Autodesk Inventor part; units mm, degrees
(part 11 of 16)
  spline S66 degree 3 poles (-38.2269, 71.8487) (-38.3811, 71.843) (-38.5356, 71.8444) (-38.6895, 71.8542) (-38.7353, 71.8572) (-38.781, 71.8608) (-38.8267, 71.8653) (-38.8695, 71.8695) (-38.9124, 71.8744) (-38.9551, 71.88) (-38.995, 71.8853) (-39.0349, 71.8912) (-39.0747, 71.8978) (-39.1117, 71.9039) (-39.1486, 71.9107) (-39.1854, 71.9181) (-39.2195, 71.9249) (-39.2534, 71.9323) (-39.2872, 71.9403) (-39.3183, 71.9476) (-39.3493, 71.9555) (-39.3802, 71.9639) (-39.4084, 71.9715) (-39.4364, 71.9796) (-39.4643, 71.9882) (-39.4895, 71.996) (-39.5146, 72.0042) (-39.5396, 72.0128) (-39.562, 72.0205) (-39.5843, 72.0284) (-39.6062, 72.0371) (-39.6255, 72.0447) (-39.6445, 72.0529) (-39.6642, 72.0604) (-39.7009, 72.0743) (-39.7403, 72.0857) (-39.7695, 72.1099) (-39.7917, 72.1282) (-39.8081, 72.1539) (-39.8266, 72.177) (-39.8422, 72.1963) (-39.8592, 72.2138) (-39.8762, 72.2316) (-39.8928, 72.2488) (-39.9093, 72.2662) (-39.9262, 72.2833) (-39.9426, 72.2999) (-39.9594, 72.3162) (-39.9764, 72.3322) (-39.9929, 72.3478) (-40.0097, 72.3632) (-40.0267, 72.3783) (-40.0434, 72.393) (-40.0602, 72.4074) (-40.0773, 72.4215) (-40.094, 72.4353) (-40.1109, 72.4488) (-40.128, 72.462) (-40.1447, 72.4749) (-40.1617, 72.4875) (-40.1789, 72.4998) (-40.1956, 72.5117) (-40.2126, 72.5234) (-40.2298, 72.5347) (-40.2466, 72.5458) (-40.2636, 72.5566) (-40.2809, 72.567) (-40.2977, 72.5772) (-40.3148, 72.587) (-40.3321, 72.5965) (-40.349, 72.6058) (-40.3661, 72.6147) (-40.3835, 72.6232) (-40.4005, 72.6316) (-40.4177, 72.6396) (-40.4351, 72.6472) (-40.4522, 72.6547) (-40.4695, 72.6617) (-40.487, 72.6683) (-40.5042, 72.6749) (-40.5217, 72.681) (-40.5393, 72.6866) (-40.5567, 72.6922) (-40.5743, 72.6973) (-40.5921, 72.7019) (-40.6097, 72.7064) (-40.6276, 72.7105) (-40.6455, 72.714) (-40.6635, 72.7175) (-40.6815, 72.7204) (-40.6997, 72.7228) (-40.718, 72.7251) (-40.7364, 72.7268) (-40.7548, 72.7279) (-40.7735, 72.7289) (-40.7923, 72.7293) (-40.811, 72.7289) (-40.8301, 72.7285) (-40.8492, 72.7273) (-40.8682, 72.7254) (-40.8877, 72.7233) (-40.9072, 72.7204) (-40.9265, 72.7166) (-40.9463, 72.7127) (-40.966, 72.7078) (-40.9854, 72.702) (-41.0054, 72.6959) (-41.0252, 72.6888) (-41.0445, 72.6807) (-41.0644, 72.6722) (-41.0839, 72.6627) (-41.1028, 72.6521) (-41.1222, 72.6411) (-41.141, 72.629) (-41.159, 72.6157) (-41.1774, 72.6022) (-41.1949, 72.5874) (-41.2116, 72.5718) (-41.2234, 72.5607) (-41.2348, 72.5491) (-41.2461, 72.5373) (-41.3001, 72.481) (-41.3504, 72.4211) (-41.4042, 72.3646) (-41.458, 72.3081) (-41.5152, 72.2549) (-41.5689, 72.1981) (-41.58, 72.1863) (-41.591, 72.1744) (-41.6016, 72.162) (-41.6164, 72.1446) (-41.6302, 72.1263) (-41.6429, 72.1073) (-41.6552, 72.0887) (-41.6664, 72.0693) (-41.6764, 72.0494) (-41.686, 72.03) (-41.6946, 72.0101) (-41.702, 71.9897) (-41.7092, 71.97) (-41.7154, 71.95) (-41.7204, 71.9297) (-41.7253, 71.91) (-41.7292, 71.8901) (-41.7321, 71.8701) (-41.735, 71.8506) (-41.7369, 71.8311) (-41.738, 71.8115) (-41.739, 71.7924) (-41.7392, 71.7732) (-41.7387, 71.7541) (-41.7381, 71.7354) (-41.7368, 71.7167) (-41.7349, 71.6981) (-41.7329, 71.6797) (-41.7303, 71.6614) (-41.727, 71.6433) (-41.7238, 71.6253) (-41.72, 71.6073) (-41.7156, 71.5896) (-41.7112, 71.5718) (-41.7063, 71.5542) (-41.7008, 71.5368) (-41.6954, 71.5193) (-41.6894, 71.502) (-41.683, 71.4848) (-41.6765, 71.4675) (-41.6695, 71.4504) (-41.6621, 71.4335) (-41.6547, 71.4164) (-41.6468, 71.3994) (-41.6385, 71.3827) (-41.63, 71.3657) (-41.6212, 71.3489) (-41.612, 71.3324) (-41.6026, 71.3155) (-41.5928, 71.2988) (-41.5827, 71.2824) (-41.5724, 71.2656) (-41.5617, 71.249) (-41.5507, 71.2327) (-41.5395, 71.216) (-41.5279, 71.1995) (-41.516, 71.1833) (-41.5038, 71.1666) (-41.4913, 71.1503) (-41.4785, 71.1341) (-41.4654, 71.1176) (-41.452, 71.1013) (-41.4383, 71.0852) (-41.4243, 71.0687) (-41.41, 71.0525) (-41.3954, 71.0366) (-41.3804, 71.0202) (-41.3652, 71.0041) (-41.3497, 70.9882) (-41.3337, 70.9719) (-41.3176, 70.9559) (-41.3011, 70.9401) (-41.2843, 70.924) (-41.2672, 70.908) (-41.2498, 70.8924) (-41.232, 70.8764) (-41.2138, 70.8608) (-41.1957, 70.8451) (-41.1772, 70.829) (-41.1588, 70.8128) (-41.1387, 70.7983) (-41.1147, 70.7809) (-41.0883, 70.7658) (-41.0689, 70.7446) (-41.0433, 70.7165) (-41.03, 70.6778) (-41.0143, 70.6418) (-41.0058, 70.6225) (-40.9967, 70.6039) (-40.9881, 70.585) (-40.9783, 70.5636) (-40.9693, 70.5417) (-40.9606, 70.5197) (-40.9508, 70.4951) (-40.9413, 70.4705) (-40.9323, 70.4457) (-40.9223, 70.4183) (-40.9128, 70.3907) (-40.9038, 70.3629) (-40.8939, 70.3325) (-40.8845, 70.302) (-40.8756, 70.2713) (-40.866, 70.2379) (-40.8569, 70.2043) (-40.8484, 70.1706) (-40.8392, 70.1343) (-40.8306, 70.0977) (-40.8227, 70.061) (-40.8141, 70.0217) (-40.8062, 69.9821) (-40.799, 69.9425) (-40.7913, 69.9001) (-40.7843, 69.8576) (-40.778, 69.815) (-40.7712, 69.7696) (-40.7653, 69.7241) (-40.7601, 69.6785) (-40.7427, 69.5253) (-40.7337, 69.371) (-40.7317, 69.2168) knots 0 0 0 0 0.065113 0.065113 0.065113 0.084473 0.084473 0.084473 0.102659 0.102659 0.102659 0.119672 0.119672 0.119672 0.135512 0.135512 0.135512 0.150178 0.150178 0.150178 0.163672 0.163672 0.163672 0.175991 0.175991 0.175991 0.187138 0.187138 0.187138 0.197111 0.197111 0.197111 0.205911 0.205911 0.205911 0.222284 0.222284 0.222284 0.234681 0.234681 0.234681 0.24506 0.24506 0.24506 0.255176 0.255176 0.255176 0.265035 0.265035 0.265035 0.274643 0.274643 0.274643 0.284008 0.284008 0.284008 0.293139 0.293139 0.293139 0.302047 0.302047 0.302047 0.310743 0.310743 0.310743 0.319241 0.319241 0.319241 0.327556 0.327556 0.327556 0.335706 0.335706 0.335706 0.343713 0.343713 0.343713 0.351599 0.351599 0.351599 0.359392 0.359392 0.359392 0.367126 0.367126 0.367126 0.374835 0.374835 0.374835 0.382562 0.382562 0.382562 0.390352 0.390352 0.390352 0.398256 0.398256 0.398256 0.406325 0.406325 0.406325 0.41461 0.41461 0.41461 0.423156 0.423156 0.423156 0.431994 0.431994 0.431994 0.441132 0.441132 0.441132 0.450548 0.450548 0.450548 0.460189 0.460189 0.460189 0.467051 0.467051 0.467051 0.5 0.5 0.5 0.532949 0.532949 0.532949 0.539811 0.539811 0.539811 0.549452 0.549452 0.549452 0.558868 0.558868 0.558868 0.568006 0.568006 0.568006 0.576844 0.576844 0.576844 0.58539 0.58539 0.58539 0.593675 0.593675 0.593675 0.601744 0.601744 0.601744 0.609648 0.609648 0.609648 0.617438 0.617438 0.617438 0.625165 0.625165 0.625165 0.632874 0.632874 0.632874 0.640608 0.640608 0.640608 0.648401 0.648401 0.648401 0.656287 0.656287 0.656287 0.664294 0.664294 0.664294 0.672444 0.672444 0.672444 0.680759 0.680759 0.680759 0.689257 0.689257 0.689257 0.697953 0.697953 0.697953 0.706861 0.706861 0.706861 0.715992 0.715992 0.715992 0.725357 0.725357 0.725357 0.734965 0.734965 0.734965 0.744824 0.744824 0.744824 0.75494 0.75494 0.75494 0.765319 0.765319 0.765319 0.777716 0.777716 0.777716 0.794089 0.794089 0.794089 0.802889 0.802889 0.802889 0.812862 0.812862 0.812862 0.824009 0.824009 0.824009 0.836328 0.836328 0.836328 0.849822 0.849822 0.849822 0.864488 0.864488 0.864488 0.880328 0.880328 0.880328 0.897341 0.897341 0.897341 0.915527 0.915527 0.915527 0.934887 0.934887 0.934887 1 1 1 1
  arc A268 (-38.2269, 71.8487) -> (-37.7508, 72.7226) centre (-45.7832, 76.5321) ccw
  spline S67 degree 3 poles (-36.8976, 76.2543) (-37.0282, 76.1723) (-37.1627, 76.0963) (-37.3009, 76.0278) (-37.342, 76.0075) (-37.3835, 75.9878) (-37.4252, 75.9688) (-37.4645, 75.951) (-37.504, 75.9338) (-37.5438, 75.9173) (-37.581, 75.9019) (-37.6185, 75.8871) (-37.6563, 75.8729) (-37.6914, 75.8598) (-37.7267, 75.8471) (-37.7623, 75.8351) (-37.7952, 75.824) (-37.8283, 75.8135) (-37.8616, 75.8035) (-37.8922, 75.7943) (-37.923, 75.7856) (-37.9539, 75.7774) (-37.9821, 75.77) (-38.0104, 75.7629) (-38.0389, 75.7565) (-38.0646, 75.7506) (-38.0905, 75.7452) (-38.1164, 75.7401) (-38.1396, 75.7355) (-38.1629, 75.7312) (-38.1862, 75.7278) (-38.2068, 75.7248) (-38.2273, 75.7224) (-38.2481, 75.719) (-38.2869, 75.7127) (-38.3266, 75.7029) (-38.3641, 75.7092) (-38.3924, 75.714) (-38.4194, 75.728) (-38.4471, 75.7388) (-38.4702, 75.7477) (-38.4938, 75.7544) (-38.5173, 75.7612) (-38.5403, 75.7679) (-38.5633, 75.7747) (-38.5864, 75.781) (-38.609, 75.7872) (-38.6316, 75.7929) (-38.6543, 75.7983) (-38.6765, 75.8035) (-38.6987, 75.8085) (-38.721, 75.813) (-38.7428, 75.8174) (-38.7646, 75.8215) (-38.7864, 75.8252) (-38.8078, 75.8288) (-38.8292, 75.8321) (-38.8506, 75.8349) (-38.8715, 75.8377) (-38.8925, 75.8401) (-38.9135, 75.8422) (-38.934, 75.8442) (-38.9546, 75.8458) (-38.9751, 75.847) (-38.9952, 75.8482) (-39.0153, 75.849) (-39.0355, 75.8494) (-39.0552, 75.8498) (-39.0749, 75.8498) (-39.0946, 75.8493) (-39.1139, 75.8489) (-39.1332, 75.8481) (-39.1524, 75.8468) (-39.1714, 75.8455) (-39.1903, 75.8439) (-39.2091, 75.8417) (-39.2277, 75.8397) (-39.2462, 75.8371) (-39.2646, 75.8341) (-39.2828, 75.8311) (-39.301, 75.8277) (-39.319, 75.8238) (-39.3369, 75.8199) (-39.3547, 75.8155) (-39.3724, 75.8106) (-39.39, 75.8057) (-39.4075, 75.8003) (-39.4247, 75.7944) (-39.442, 75.7885) (-39.4592, 75.782) (-39.4761, 75.7749) (-39.4931, 75.7678) (-39.5099, 75.7601) (-39.5264, 75.7517) (-39.5431, 75.7433) (-39.5595, 75.7342) (-39.5755, 75.7246) (-39.5919, 75.7147) (-39.6078, 75.7041) (-39.6233, 75.6929) (-39.6392, 75.6813) (-39.6546, 75.6691) (-39.6694, 75.6562) (-39.6846, 75.6429) (-39.6992, 75.6288) (-39.7131, 75.614) (-39.7274, 75.5988) (-39.741, 75.5827) (-39.7536, 75.566) (-39.7667, 75.5488) (-39.7788, 75.5308) (-39.7898, 75.5121) (-39.8012, 75.4929) (-39.8114, 75.473) (-39.8203, 75.4526) (-39.8295, 75.4316) (-39.8373, 75.4101) (-39.8439, 75.3882) (-39.8486, 75.3726) (-39.8526, 75.3569) (-39.8565, 75.3411) (-39.8751, 75.2653) (-39.8888, 75.1883) (-39.9071, 75.1125) (-39.9254, 75.0366) (-39.9484, 74.9619) (-39.9665, 74.886) (-39.9702, 74.8702) (-39.9738, 74.8543) (-39.9767, 74.8383) (-39.9808, 74.8158) (-39.9837, 74.7931) (-39.9852, 74.7703) (-39.9865, 74.748) (-39.9865, 74.7257) (-39.9852, 74.7034) (-39.9839, 74.6818) (-39.9813, 74.6602) (-39.9776, 74.6389) (-39.974, 74.6182) (-39.9693, 74.5978) (-39.9635, 74.5777) (-39.9579, 74.5582) (-39.9513, 74.539) (-39.9438, 74.5202) (-39.9366, 74.502) (-39.9285, 74.4841) (-39.9196, 74.4665) (-39.9109, 74.4495) (-39.9016, 74.4328) (-39.8915, 74.4165) (-39.8817, 74.4006) (-39.8712, 74.385) (-39.8602, 74.3699) (-39.8493, 74.355) (-39.8379, 74.3405) (-39.826, 74.3264) (-39.8142, 74.3124) (-39.802, 74.2988) (-39.7893, 74.2856) (-39.7766, 74.2724) (-39.7635, 74.2596) (-39.7501, 74.2472) (-39.7366, 74.2348) (-39.7228, 74.2228) (-39.7086, 74.2112) (-39.6944, 74.1994) (-39.6798, 74.1881) (-39.6649, 74.1771) (-39.6499, 74.166) (-39.6346, 74.1553) (-39.619, 74.145) (-39.6032, 74.1345) (-39.5872, 74.1244) (-39.5709, 74.1146) (-39.5544, 74.1047) (-39.5376, 74.0951) (-39.5206, 74.086) (-39.5033, 74.0766) (-39.4857, 74.0676) (-39.468, 74.0589) (-39.45, 74.0501) (-39.4317, 74.0416) (-39.4133, 74.0335) (-39.3944, 74.0252) (-39.3754, 74.0172) (-39.3562, 74.0096) (-39.3366, 74.0019) (-39.3169, 73.9945) (-39.297, 73.9874) (-39.2766, 73.9801) (-39.2561, 73.9733) (-39.2355, 73.9667) (-39.2143, 73.96) (-39.193, 73.9537) (-39.1717, 73.9477) (-39.1498, 73.9416) (-39.1277, 73.9358) (-39.1056, 73.9304) (-39.083, 73.9248) (-39.0602, 73.9195) (-39.0373, 73.9147) (-39.0139, 73.9098) (-38.9903, 73.9054) (-38.9668, 73.9008) (-38.9427, 73.8961) (-38.9187, 73.8913) (-38.894, 73.8887) (-38.8646, 73.8856) (-38.8341, 73.8858) (-38.8067, 73.8771) (-38.7705, 73.8657) (-38.7396, 73.8387) (-38.708, 73.8154) (-38.691, 73.8029) (-38.6738, 73.7914) (-38.6569, 73.7794) (-38.6378, 73.7657) (-38.619, 73.7512) (-38.6005, 73.7365) (-38.5797, 73.7202) (-38.5592, 73.7036) (-38.539, 73.6866) (-38.5166, 73.6679) (-38.4946, 73.6487) (-38.4729, 73.6292) (-38.4491, 73.6078) (-38.4257, 73.586) (-38.4027, 73.5638) (-38.3776, 73.5398) (-38.353, 73.5152) (-38.3288, 73.4903) (-38.3026, 73.4634) (-38.2769, 73.4361) (-38.2517, 73.4083) (-38.2246, 73.3785) (-38.198, 73.3482) (-38.1719, 73.3174) (-38.144, 73.2846) (-38.1167, 73.2513) (-38.0899, 73.2175) (-38.0614, 73.1816) (-38.0336, 73.1452) (-38.0063, 73.1083) (-37.9146, 72.9843) (-37.8296, 72.8552) (-37.7508, 72.7226) knots 0 0 0 0 0.065113 0.065113 0.065113 0.084473 0.084473 0.084473 0.102659 0.102659 0.102659 0.119672 0.119672 0.119672 0.135512 0.135512 0.135512 0.150178 0.150178 0.150178 0.163672 0.163672 0.163672 0.175991 0.175991 0.175991 0.187138 0.187138 0.187138 0.197111 0.197111 0.197111 0.205911 0.205911 0.205911 0.222284 0.222284 0.222284 0.234681 0.234681 0.234681 0.24506 0.24506 0.24506 0.255176 0.255176 0.255176 0.265035 0.265035 0.265035 0.274643 0.274643 0.274643 0.284008 0.284008 0.284008 0.293139 0.293139 0.293139 0.302047 0.302047 0.302047 0.310743 0.310743 0.310743 0.319241 0.319241 0.319241 0.327556 0.327556 0.327556 0.335706 0.335706 0.335706 0.343713 0.343713 0.343713 0.351599 0.351599 0.351599 0.359392 0.359392 0.359392 0.367126 0.367126 0.367126 0.374835 0.374835 0.374835 0.382562 0.382562 0.382562 0.390352 0.390352 0.390352 0.398256 0.398256 0.398256 0.406325 0.406325 0.406325 0.41461 0.41461 0.41461 0.423156 0.423156 0.423156 0.431994 0.431994 0.431994 0.441132 0.441132 0.441132 0.450548 0.450548 0.450548 0.460189 0.460189 0.460189 0.467051 0.467051 0.467051 0.5 0.5 0.5 0.532949 0.532949 0.532949 0.539811 0.539811 0.539811 0.549452 0.549452 0.549452 0.558868 0.558868 0.558868 0.568006 0.568006 0.568006 0.576844 0.576844 0.576844 0.58539 0.58539 0.58539 0.593675 0.593675 0.593675 0.601744 0.601744 0.601744 0.609648 0.609648 0.609648 0.617438 0.617438 0.617438 0.625165 0.625165 0.625165 0.632874 0.632874 0.632874 0.640608 0.640608 0.640608 0.648401 0.648401 0.648401 0.656287 0.656287 0.656287 0.664294 0.664294 0.664294 0.672444 0.672444 0.672444 0.680759 0.680759 0.680759 0.689257 0.689257 0.689257 0.697953 0.697953 0.697953 0.706861 0.706861 0.706861 0.715992 0.715992 0.715992 0.725357 0.725357 0.725357 0.734965 0.734965 0.734965 0.744824 0.744824 0.744824 0.75494 0.75494 0.75494 0.765319 0.765319 0.765319 0.777716 0.777716 0.777716 0.794089 0.794089 0.794089 0.802889 0.802889 0.802889 0.812862 0.812862 0.812862 0.824009 0.824009 0.824009 0.836328 0.836328 0.836328 0.849822 0.849822 0.849822 0.864488 0.864488 0.864488 0.880328 0.880328 0.880328 0.897341 0.897341 0.897341 0.915527 0.915527 0.915527 0.934887 0.934887 0.934887 1 1 1 1
  arc A269 (-36.8976, 76.2543) -> (-36.9222, 77.2492) centre (-45.7832, 76.5321) ccw
  spline S68 degree 3 poles (-37.9491, 80.7344) (-38.0213, 80.598) (-38.0997, 80.4649) (-38.1852, 80.3365) (-38.2106, 80.2983) (-38.2366, 80.2606) (-38.2633, 80.2233) (-38.2884, 80.1882) (-38.314, 80.1536) (-38.3403, 80.1194) (-38.3648, 80.0874) (-38.3899, 80.0559) (-38.4155, 80.0247) (-38.4393, 79.9958) (-38.4636, 79.9672) (-38.4884, 79.939) (-38.5113, 79.9129) (-38.5347, 79.8872) (-38.5586, 79.8619) (-38.5805, 79.8386) (-38.6028, 79.8157) (-38.6254, 79.7932) (-38.6462, 79.7726) (-38.6672, 79.7524) (-38.6886, 79.7325) (-38.708, 79.7146) (-38.7276, 79.697) (-38.7475, 79.6796) (-38.7654, 79.6641) (-38.7834, 79.6487) (-38.8018, 79.6341) (-38.8181, 79.6212) (-38.8347, 79.6089) (-38.8511, 79.5955) (-38.8815, 79.5707) (-38.911, 79.5423) (-38.9466, 79.529) (-38.9735, 79.519) (-39.0039, 79.5177) (-39.0332, 79.5131) (-39.0578, 79.5093) (-39.0815, 79.5033) (-39.1053, 79.4974) (-39.1285, 79.4917) (-39.1519, 79.4861) (-39.1751, 79.4801) (-39.1977, 79.4742) (-39.2201, 79.4678) (-39.2425, 79.4611) (-39.2643, 79.4545) (-39.286, 79.4477) (-39.3076, 79.4405) (-39.3287, 79.4334) (-39.3496, 79.426) (-39.3704, 79.4183) (-39.3906, 79.4108) (-39.4108, 79.4029) (-39.4308, 79.3946) (-39.4503, 79.3866) (-39.4697, 79.3782) (-39.4889, 79.3695) (-39.5076, 79.361) (-39.5262, 79.3521) (-39.5447, 79.3428) (-39.5627, 79.3338) (-39.5805, 79.3245) (-39.5981, 79.3147) (-39.6154, 79.3052) (-39.6324, 79.2954) (-39.6493, 79.2851) (-39.6658, 79.2751) (-39.6821, 79.2647) (-39.6981, 79.254) (-39.7139, 79.2435) (-39.7294, 79.2326) (-39.7447, 79.2213) (-39.7597, 79.2102) (-39.7745, 79.1988) (-39.7889, 79.1869) (-39.8032, 79.1752) (-39.8172, 79.1632) (-39.8309, 79.1508) (-39.8445, 79.1385) (-39.8577, 79.1258) (-39.8705, 79.1127) (-39.8833, 79.0997) (-39.8957, 79.0863) (-39.9077, 79.0725) (-39.9198, 79.0587) (-39.9313, 79.0445) (-39.9424, 79.0299) (-39.9536, 79.0152) (-39.9643, 79.0002) (-39.9744, 78.9847) (-39.9847, 78.9691) (-39.9944, 78.953) (-40.0034, 78.9366) (-40.0126, 78.9199) (-40.0212, 78.9027) (-40.0289, 78.8853) (-40.0369, 78.8673) (-40.0442, 78.8491) (-40.0505, 78.8305) (-40.057, 78.8113) (-40.0627, 78.7918) (-40.0673, 78.7721) (-40.0721, 78.7517) (-40.0758, 78.7311) (-40.0784, 78.7103) (-40.081, 78.6888) (-40.0825, 78.6671) (-40.0827, 78.6455) (-40.083, 78.6232) (-40.0819, 78.6008) (-40.0794, 78.5786) (-40.0769, 78.5559) (-40.0728, 78.5334) (-40.0676, 78.5112) (-40.0639, 78.4953) (-40.0596, 78.4796) (-40.055, 78.464) (-40.0332, 78.3891) (-40.0066, 78.3156) (-39.9845, 78.2407) (-39.9624, 78.1659) (-39.945, 78.0897) (-39.9227, 78.0149) (-39.918, 77.9993) (-39.9132, 77.9838) (-39.9077, 77.9685) (-39.9001, 77.947) (-39.8912, 77.9258) (-39.881, 77.9054) (-39.8711, 77.8854) (-39.8599, 77.866) (-39.8476, 77.8474) (-39.8357, 77.8293) (-39.8227, 77.8119) (-39.8088, 77.7953) (-39.7953, 77.7793) (-39.781, 77.7639) (-39.7659, 77.7494) (-39.7514, 77.7353) (-39.7361, 77.722) (-39.7202, 77.7095) (-39.7048, 77.6973) (-39.6888, 77.6858) (-39.6724, 77.6751) (-39.6564, 77.6647) (-39.6399, 77.6549) (-39.6231, 77.6458) (-39.6066, 77.6369) (-39.5897, 77.6287) (-39.5726, 77.6211) (-39.5557, 77.6136) (-39.5386, 77.6067) (-39.5212, 77.6005) (-39.504, 77.5942) (-39.4866, 77.5886) (-39.469, 77.5835) (-39.4515, 77.5784) (-39.4338, 77.5739) (-39.4159, 77.5699) (-39.3981, 77.5659) (-39.3801, 77.5624) (-39.362, 77.5594) (-39.3438, 77.5564) (-39.3255, 77.5538) (-39.3071, 77.5518) (-39.2886, 77.5497) (-39.2699, 77.5481) (-39.2513, 77.5469) (-39.2324, 77.5457) (-39.2134, 77.545) (-39.1944, 77.5447) (-39.1751, 77.5443) (-39.1558, 77.5445) (-39.1365, 77.545) (-39.1168, 77.5455) (-39.0972, 77.5465) (-39.0775, 77.5479) (-39.0574, 77.5492) (-39.0374, 77.551) (-39.0173, 77.5532) (-38.9969, 77.5555) (-38.9764, 77.5581) (-38.956, 77.5611) (-38.9352, 77.5642) (-38.9143, 77.5676) (-38.8936, 77.5714) (-38.8723, 77.5754) (-38.8511, 77.5797) (-38.83, 77.5843) (-38.8083, 77.5891) (-38.7867, 77.5942) (-38.7652, 77.5997) (-38.7432, 77.6054) (-38.7212, 77.6114) (-38.6994, 77.6177) (-38.6769, 77.6242) (-38.6546, 77.631) (-38.6324, 77.6383) (-38.6096, 77.6458) (-38.587, 77.6538) (-38.5644, 77.6616) (-38.5411, 77.6695) (-38.5179, 77.6773) (-38.4953, 77.6875) (-38.4682, 77.6995) (-38.4419, 77.7149) (-38.4139, 77.7211) (-38.3768, 77.7293) (-38.3366, 77.7214) (-38.2976, 77.717) (-38.2766, 77.7147) (-38.256, 77.7133) (-38.2353, 77.7113) (-38.2119, 77.709) (-38.1884, 77.7059) (-38.165, 77.7025) (-38.1388, 77.6987) (-38.1127, 77.6945) (-38.0867, 77.69) (-38.058, 77.6849) (-38.0294, 77.6793) (-38.0008, 77.6732) (-37.9695, 77.6666) (-37.9384, 77.6595) (-37.9073, 77.6518) (-37.8736, 77.6435) (-37.84, 77.6345) (-37.8066, 77.6251) (-37.7705, 77.6148) (-37.7346, 77.604) (-37.6988, 77.5926) (-37.6604, 77.5803) (-37.6222, 77.5673) (-37.5843, 77.5538) (-37.5437, 77.5393) (-37.5034, 77.5241) (-37.4633, 77.5082) (-37.4207, 77.4914) (-37.3783, 77.4737) (-37.3363, 77.4555) (-37.1948, 77.3939) (-37.0568, 77.3246) (-36.9222, 77.2492) knots 0 0 0 0 0.065113 0.065113 0.065113 0.084473 0.084473 0.084473 0.102659 0.102659 0.102659 0.119672 0.119672 0.119672 0.135512 0.135512 0.135512 0.150178 0.150178 0.150178 0.163672 0.163672 0.163672 0.175991 0.175991 0.175991 0.187138 0.187138 0.187138 0.197111 0.197111 0.197111 0.205911 0.205911 0.205911 0.222284 0.222284 0.222284 0.234681 0.234681 0.234681 0.24506 0.24506 0.24506 0.255176 0.255176 0.255176 0.265035 0.265035 0.265035 0.274643 0.274643 0.274643 0.284008 0.284008 0.284008 0.293139 0.293139 0.293139 0.302047 0.302047 0.302047 0.310743 0.310743 0.310743 0.319241 0.319241 0.319241 0.327556 0.327556 0.327556 0.335706 0.335706 0.335706 0.343713 0.343713 0.343713 0.351599 0.351599 0.351599 0.359392 0.359392 0.359392 0.367126 0.367126 0.367126 0.374835 0.374835 0.374835 0.382562 0.382562 0.382562 0.390352 0.390352 0.390352 0.398256 0.398256 0.398256 0.406325 0.406325 0.406325 0.41461 0.41461 0.41461 0.423156 0.423156 0.423156 0.431994 0.431994 0.431994 0.441132 0.441132 0.441132 0.450548 0.450548 0.450548 0.460189 0.460189 0.460189 0.467051 0.467051 0.467051 0.5 0.5 0.5 0.532949 0.532949 0.532949 0.539811 0.539811 0.539811 0.549452 0.549452 0.549452 0.558868 0.558868 0.558868 0.568006 0.568006 0.568006 0.576844 0.576844 0.576844 0.58539 0.58539 0.58539 0.593675 0.593675 0.593675 0.601744 0.601744 0.601744 0.609648 0.609648 0.609648 0.617438 0.617438 0.617438 0.625165 0.625165 0.625165 0.632874 0.632874 0.632874 0.640608 0.640608 0.640608 0.648401 0.648401 0.648401 0.656287 0.656287 0.656287 0.664294 0.664294 0.664294 0.672444 0.672444 0.672444 0.680759 0.680759 0.680759 0.689257 0.689257 0.689257 0.697953 0.697953 0.697953 0.706861 0.706861 0.706861 0.715992 0.715992 0.715992 0.725357 0.725357 0.725357 0.734965 0.734965 0.734965 0.744824 0.744824 0.744824 0.75494 0.75494 0.75494 0.765319 0.765319 0.765319 0.777716 0.777716 0.777716 0.794089 0.794089 0.794089 0.802889 0.802889 0.802889 0.812862 0.812862 0.812862 0.824009 0.824009 0.824009 0.836328 0.836328 0.836328 0.849822 0.849822 0.849822 0.864488 0.864488 0.864488 0.880328 0.880328 0.880328 0.897341 0.897341 0.897341 0.915527 0.915527 0.915527 0.934887 0.934887 0.934887 1 1 1 1
  arc A270 (-37.9491, 80.7344) -> (-38.4679, 81.5836) centre (-45.7832, 76.5321) ccw
  spline S69 degree 3 poles (-41.0998, 84.0884) (-41.0941, 83.9343) (-41.0955, 83.7798) (-41.1053, 83.6258) (-41.1082, 83.5801) (-41.1119, 83.5344) (-41.1164, 83.4887) (-41.1206, 83.4458) (-41.1254, 83.403) (-41.1311, 83.3603) (-41.1363, 83.3203) (-41.1422, 83.2805) (-41.1488, 83.2407) (-41.155, 83.2037) (-41.1617, 83.1668) (-41.1691, 83.13) (-41.176, 83.0959) (-41.1834, 83.0619) (-41.1914, 83.0281) (-41.1987, 82.997) (-41.2065, 82.966) (-41.2149, 82.9352) (-41.2226, 82.907) (-41.2307, 82.879) (-41.2393, 82.8511) (-41.2471, 82.8259) (-41.2553, 82.8008) (-41.2639, 82.7758) (-41.2715, 82.7534) (-41.2795, 82.7311) (-41.2881, 82.7092) (-41.2958, 82.6899) (-41.304, 82.6709) (-41.3115, 82.6512) (-41.3254, 82.6145) (-41.3368, 82.5751) (-41.3609, 82.5458) (-41.3793, 82.5237) (-41.4049, 82.5073) (-41.4281, 82.4887) (-41.4474, 82.4732) (-41.4649, 82.4561) (-41.4826, 82.4391) (-41.4999, 82.4226) (-41.5173, 82.4061) (-41.5344, 82.3892) (-41.551, 82.3728) (-41.5672, 82.356) (-41.5833, 82.339) (-41.5989, 82.3225) (-41.6142, 82.3057) (-41.6293, 82.2886) (-41.644, 82.272) (-41.6585, 82.2552) (-41.6726, 82.2381) (-41.6864, 82.2214) (-41.6999, 82.2045) (-41.7131, 82.1873) (-41.726, 82.1706) (-41.7386, 82.1537) (-41.7508, 82.1365) (-41.7628, 82.1198) (-41.7745, 82.1028) (-41.7858, 82.0856) (-41.7969, 82.0688) (-41.8077, 82.0517) (-41.8181, 82.0345) (-41.8282, 82.0176) (-41.8381, 82.0006) (-41.8475, 81.9833) (-41.8568, 81.9664) (-41.8658, 81.9492) (-41.8743, 81.9319) (-41.8827, 81.9149) (-41.8907, 81.8977) (-41.8983, 81.8803) (-41.9057, 81.8632) (-41.9128, 81.8459) (-41.9194, 81.8284) (-41.9259, 81.8111) (-41.9321, 81.7937) (-41.9377, 81.7761) (-41.9433, 81.7587) (-41.9484, 81.7411) (-41.9529, 81.7233) (-41.9575, 81.7056) (-41.9616, 81.6878) (-41.9651, 81.6699) (-41.9686, 81.6519) (-41.9715, 81.6338) (-41.9738, 81.6157) (-41.9762, 81.5974) (-41.9779, 81.579) (-41.9789, 81.5605) (-41.98, 81.5418) (-41.9804, 81.5231) (-41.98, 81.5044) (-41.9796, 81.4853) (-41.9784, 81.4662) (-41.9764, 81.4471) (-41.9744, 81.4276) (-41.9715, 81.4082) (-41.9677, 81.3889) (-41.9638, 81.369) (-41.9589, 81.3494) (-41.953, 81.33) (-41.947, 81.3099) (-41.9399, 81.2902) (-41.9317, 81.2709) (-41.9233, 81.2509) (-41.9138, 81.2315) (-41.9031, 81.2126) (-41.8922, 81.1931) (-41.8801, 81.1743) (-41.8668, 81.1564) (-41.8533, 81.138) (-41.8385, 81.1205) (-41.8229, 81.1038) (-41.8117, 81.092) (-41.8001, 81.0806) (-41.7884, 81.0693) (-41.732, 81.0153) (-41.6722, 80.965) (-41.6157, 80.9112) (-41.5592, 80.8574) (-41.5059, 80.8001) (-41.4492, 80.7465) (-41.4374, 80.7353) (-41.4254, 80.7243) (-41.4131, 80.7138) (-41.3957, 80.699) (-41.3774, 80.6851) (-41.3584, 80.6725) (-41.3398, 80.6602) (-41.3204, 80.649) (-41.3004, 80.639) (-41.2811, 80.6293) (-41.2611, 80.6207) (-41.2408, 80.6133) (-41.2211, 80.6061) (-41.2011, 80.6) (-41.1807, 80.595) (-41.1611, 80.5901) (-41.1412, 80.5862) (-41.1211, 80.5832) (-41.1017, 80.5804) (-41.0822, 80.5785) (-41.0625, 80.5774) (-41.0435, 80.5764) (-41.0243, 80.5761) (-41.0052, 80.5767) (-40.9865, 80.5772) (-40.9678, 80.5785) (-40.9492, 80.5805) (-40.9308, 80.5825) (-40.9125, 80.5851) (-40.8944, 80.5883) (-40.8763, 80.5915) (-40.8584, 80.5954) (-40.8406, 80.5998) (-40.8229, 80.6041) (-40.8053, 80.6091) (-40.7879, 80.6145) (-40.7704, 80.62) (-40.7531, 80.6259) (-40.7359, 80.6324) (-40.7186, 80.6389) (-40.7015, 80.6458) (-40.6846, 80.6532) (-40.6675, 80.6607) (-40.6505, 80.6686) (-40.6338, 80.6769) (-40.6168, 80.6853) (-40.6, 80.6942) (-40.5834, 80.7034) (-40.5666, 80.7128) (-40.5499, 80.7225) (-40.5334, 80.7326) (-40.5167, 80.743) (-40.5001, 80.7536) (-40.4838, 80.7646) (-40.4671, 80.7759) (-40.4506, 80.7875) (-40.4343, 80.7994) (-40.4177, 80.8115) (-40.4013, 80.824) (-40.3852, 80.8368) (-40.3686, 80.8499) (-40.3523, 80.8633) (-40.3363, 80.877) (-40.3198, 80.8911) (-40.3036, 80.9054) (-40.2876, 80.92) (-40.2713, 80.9349) (-40.2551, 80.9502) (-40.2393, 80.9657) (-40.223, 80.9816) (-40.207, 80.9978) (-40.1912, 81.0142) (-40.175, 81.0311) (-40.1591, 81.0481) (-40.1435, 81.0655) (-40.1275, 81.0834) (-40.1119, 81.1016) (-40.0962, 81.1197) (-40.0801, 81.1382) (-40.0639, 81.1565) (-40.0493, 81.1766) (-40.0319, 81.2006) (-40.0169, 81.2271) (-39.9956, 81.2465) (-39.9676, 81.2721) (-39.9289, 81.2854) (-39.8929, 81.3011) (-39.8736, 81.3095) (-39.855, 81.3187) (-39.8361, 81.3273) (-39.8147, 81.337) (-39.7928, 81.346) (-39.7708, 81.3548) (-39.7462, 81.3646) (-39.7216, 81.374) (-39.6968, 81.3831) (-39.6694, 81.3931) (-39.6418, 81.4025) (-39.614, 81.4116) (-39.5836, 81.4215) (-39.553, 81.4308) (-39.5223, 81.4397) (-39.4889, 81.4494) (-39.4554, 81.4584) (-39.4217, 81.467) (-39.3853, 81.4762) (-39.3488, 81.4847) (-39.3121, 81.4927) (-39.2727, 81.5013) (-39.2332, 81.5091) (-39.1936, 81.5164) (-39.1512, 81.5241) (-39.1087, 81.5311) (-39.066, 81.5374) (-39.0207, 81.5441) (-38.9752, 81.55) (-38.9296, 81.5552) (-38.7763, 81.5727) (-38.6221, 81.5817) (-38.4679, 81.5836) knots 0 0 0 0 0.065113 0.065113 0.065113 0.084473 0.084473 0.084473 0.102659 0.102659 0.102659 0.119672 0.119672 0.119672 0.135512 0.135512 0.135512 0.150178 0.150178 0.150178 0.163672 0.163672 0.163672 0.175991 0.175991 0.175991 0.187138 0.187138 0.187138 0.197111 0.197111 0.197111 0.205911 0.205911 0.205911 0.222284 0.222284 0.222284 0.234681 0.234681 0.234681 0.24506 0.24506 0.24506 0.255176 0.255176 0.255176 0.265035 0.265035 0.265035 0.274643 0.274643 0.274643 0.284008 0.284008 0.284008 0.293139 0.293139 0.293139 0.302047 0.302047 0.302047 0.310743 0.310743 0.310743 0.319241 0.319241 0.319241 0.327556 0.327556 0.327556 0.335706 0.335706 0.335706 0.343713 0.343713 0.343713 0.351599 0.351599 0.351599 0.359392 0.359392 0.359392 0.367126 0.367126 0.367126 0.374835 0.374835 0.374835 0.382562 0.382562 0.382562 0.390352 0.390352 0.390352 0.398256 0.398256 0.398256 0.406325 0.406325 0.406325 0.41461 0.41461 0.41461 0.423156 0.423156 0.423156 0.431994 0.431994 0.431994 0.441132 0.441132 0.441132 0.450548 0.450548 0.450548 0.460189 0.460189 0.460189 0.467051 0.467051 0.467051 0.5 0.5 0.5 0.532949 0.532949 0.532949 0.539811 0.539811 0.539811 0.549452 0.549452 0.549452 0.558868 0.558868 0.558868 0.568006 0.568006 0.568006 0.576844 0.576844 0.576844 0.58539 0.58539 0.58539 0.593675 0.593675 0.593675 0.601744 0.601744 0.601744 0.609648 0.609648 0.609648 0.617438 0.617438 0.617438 0.625165 0.625165 0.625165 0.632874 0.632874 0.632874 0.640608 0.640608 0.640608 0.648401 0.648401 0.648401 0.656287 0.656287 0.656287 0.664294 0.664294 0.664294 0.672444 0.672444 0.672444 0.680759 0.680759 0.680759 0.689257 0.689257 0.689257 0.697953 0.697953 0.697953 0.706861 0.706861 0.706861 0.715992 0.715992 0.715992 0.725357 0.725357 0.725357 0.734965 0.734965 0.734965 0.744824 0.744824 0.744824 0.75494 0.75494 0.75494 0.765319 0.765319 0.765319 0.777716 0.777716 0.777716 0.794089 0.794089 0.794089 0.802889 0.802889 0.802889 0.812862 0.812862 0.812862 0.824009 0.824009 0.824009 0.836328 0.836328 0.836328 0.849822 0.849822 0.849822 0.864488 0.864488 0.864488 0.880328 0.880328 0.880328 0.897341 0.897341 0.897341 0.915527 0.915527 0.915527 0.934887 0.934887 0.934887 1 1 1 1
  arc A271 (-41.0998, 84.0884) -> (-41.9737, 84.5645) centre (-45.7832, 76.5321) ccw
  spline S70 degree 3 poles (-45.5054, 85.4178) (-45.4234, 85.2871) (-45.3473, 85.1527) (-45.2789, 85.0144) (-45.2585, 84.9733) (-45.2388, 84.9319) (-45.2199, 84.8901) (-45.2021, 84.8509) (-45.1849, 84.8114) (-45.1684, 84.7716) (-45.153, 84.7343) (-45.1382, 84.6968) (-45.124, 84.6591) (-45.1108, 84.624) (-45.0982, 84.5886) (-45.0862, 84.5531) (-45.0751, 84.5201) (-45.0645, 84.487) (-45.0545, 84.4538) (-45.0453, 84.4232) (-45.0367, 84.3924) (-45.0285, 84.3615) (-45.021, 84.3333) (-45.014, 84.3049) (-45.0075, 84.2765) (-45.0017, 84.2507) (-44.9963, 84.2249) (-44.9912, 84.199) (-44.9866, 84.1757) (-44.9823, 84.1524) (-44.9789, 84.1292) (-44.9758, 84.1086) (-44.9735, 84.0881) (-44.9701, 84.0672) (-44.9638, 84.0285) (-44.9539, 83.9887) (-44.9603, 83.9513) (-44.9651, 83.9229) (-44.9791, 83.8959) (-44.9898, 83.8683) (-44.9988, 83.8452) (-45.0055, 83.8216) (-45.0123, 83.798) (-45.0189, 83.7751) (-45.0258, 83.7521) (-45.0321, 83.7289) (-45.0383, 83.7064) (-45.044, 83.6838) (-45.0494, 83.661) (-45.0546, 83.6389) (-45.0595, 83.6166) (-45.0641, 83.5943) (-45.0685, 83.5726) (-45.0726, 83.5508) (-45.0763, 83.5289) (-45.0799, 83.5076) (-45.0831, 83.4862) (-45.086, 83.4648) (-45.0888, 83.4438) (-45.0912, 83.4229) (-45.0933, 83.4019) (-45.0953, 83.3814) (-45.0969, 83.3608) (-45.0981, 83.3402) (-45.0993, 83.3202) (-45.1001, 83.3) (-45.1005, 83.2799) (-45.1008, 83.2602) (-45.1008, 83.2405) (-45.1004, 83.2208) (-45.1, 83.2015) (-45.0991, 83.1822) (-45.0979, 83.1629) (-45.0966, 83.144) (-45.0949, 83.1251) (-45.0928, 83.1063) (-45.0907, 83.0877) (-45.0882, 83.0692) (-45.0852, 83.0507) (-45.0822, 83.0325) (-45.0788, 83.0144) (-45.0749, 82.9963) (-45.071, 82.9784) (-45.0666, 82.9606) (-45.0617, 82.943) (-45.0568, 82.9254) (-45.0514, 82.9079) (-45.0455, 82.8906) (-45.0395, 82.8733) (-45.033, 82.8562) (-45.026, 82.8393) (-45.0188, 82.8223) (-45.0111, 82.8055) (-45.0028, 82.789) (-44.9944, 82.7723) (-44.9853, 82.7559) (-44.9756, 82.7399) (-44.9657, 82.7235) (-44.9552, 82.7075) (-44.9439, 82.6921) (-44.9324, 82.6762) (-44.9202, 82.6608) (-44.9073, 82.646) (-44.8939, 82.6307) (-44.8799, 82.6161) (-44.8651, 82.6023) (-44.8498, 82.5879) (-44.8338, 82.5744) (-44.8171, 82.5618) (-44.7998, 82.5487) (-44.7818, 82.5366) (-44.7632, 82.5256) (-44.744, 82.5142) (-44.7241, 82.504) (-44.7036, 82.495) (-44.6827, 82.4859) (-44.6612, 82.4781) (-44.6393, 82.4715) (-44.6237, 82.4668) (-44.608, 82.4627) (-44.5922, 82.4589) (-44.5164, 82.4403) (-44.4394, 82.4266) (-44.3636, 82.4083) (-44.2877, 82.39) (-44.213, 82.367) (-44.137, 82.3489) (-44.1212, 82.3451) (-44.1054, 82.3416) (-44.0894, 82.3386) (-44.0669, 82.3345) (-44.0442, 82.3316) (-44.0214, 82.3302) (-43.9991, 82.3288) (-43.9767, 82.3288) (-43.9544, 82.3302) (-43.9328, 82.3315) (-43.9113, 82.334) (-43.89, 82.3378) (-43.8693, 82.3414) (-43.8489, 82.3461) (-43.8288, 82.3519) (-43.8093, 82.3575) (-43.7901, 82.3641) (-43.7713, 82.3715) (-43.753, 82.3788) (-43.7351, 82.3869) (-43.7176, 82.3958) (-43.7006, 82.4044) (-43.6839, 82.4138) (-43.6676, 82.4238) (-43.6517, 82.4337) (-43.6361, 82.4441) (-43.621, 82.4552) (-43.6061, 82.466) (-43.5915, 82.4774) (-43.5774, 82.4893) (-43.5634, 82.5011) (-43.5498, 82.5134) (-43.5366, 82.5261) (-43.5235, 82.5388) (-43.5107, 82.5518) (-43.4983, 82.5653) (-43.4859, 82.5787) (-43.4739, 82.5926) (-43.4622, 82.6067) (-43.4505, 82.621) (-43.4392, 82.6356) (-43.4282, 82.6504) (-43.4171, 82.6655) (-43.4064, 82.6808) (-43.3961, 82.6963) (-43.3856, 82.7121) (-43.3755, 82.7282) (-43.3657, 82.7445) (-43.3558, 82.761) (-43.3462, 82.7778) (-43.337, 82.7948) (-43.3276, 82.8121) (-43.3186, 82.8296) (-43.31, 82.8473) (-43.3012, 82.8654) (-43.2927, 82.8837) (-43.2846, 82.9021) (-43.2763, 82.921) (-43.2683, 82.94) (-43.2607, 82.9591) (-43.2529, 82.9787) (-43.2455, 82.9985) (-43.2385, 83.0184) (-43.2312, 83.0388) (-43.2243, 83.0593) (-43.2178, 83.0799) (-43.2111, 83.1011) (-43.2048, 83.1223) (-43.1988, 83.1437) (-43.1927, 83.1656) (-43.1869, 83.1876) (-43.1814, 83.2097) (-43.1758, 83.2324) (-43.1706, 83.2552) (-43.1658, 83.278) (-43.1609, 83.3015) (-43.1565, 83.3251) (-43.1519, 83.3486) (-43.1472, 83.3727) (-43.1424, 83.3967) (-43.1398, 83.4213) (-43.1367, 83.4508) (-43.1369, 83.4813) (-43.1282, 83.5087) (-43.1167, 83.5449) (-43.0898, 83.5757) (-43.0665, 83.6073) (-43.054, 83.6243) (-43.0425, 83.6415) (-43.0304, 83.6584) (-43.0167, 83.6776) (-43.0023, 83.6963) (-42.9876, 83.7149) (-42.9712, 83.7357) (-42.9546, 83.7562) (-42.9377, 83.7764) (-42.9189, 83.7988) (-42.8998, 83.8208) (-42.8802, 83.8425) (-42.8589, 83.8662) (-42.8371, 83.8896) (-42.8149, 83.9127) (-42.7908, 83.9377) (-42.7663, 83.9623) (-42.7414, 83.9866) (-42.7145, 84.0127) (-42.6871, 84.0384) (-42.6594, 84.0637) (-42.6295, 84.0908) (-42.5992, 84.1174) (-42.5685, 84.1434) (-42.5357, 84.1713) (-42.5024, 84.1987) (-42.4686, 84.2254) (-42.4327, 84.2539) (-42.3962, 84.2818) (-42.3594, 84.3091) (-42.2353, 84.4008) (-42.1063, 84.4857) (-41.9737, 84.5645) knots 0 0 0 0 0.065113 0.065113 0.065113 0.084473 0.084473 0.084473 0.102659 0.102659 0.102659 0.119672 0.119672 0.119672 0.135512 0.135512 0.135512 0.150178 0.150178 0.150178 0.163672 0.163672 0.163672 0.175991 0.175991 0.175991 0.187138 0.187138 0.187138 0.197111 0.197111 0.197111 0.205911 0.205911 0.205911 0.222284 0.222284 0.222284 0.234681 0.234681 0.234681 0.24506 0.24506 0.24506 0.255176 0.255176 0.255176 0.265035 0.265035 0.265035 0.274643 0.274643 0.274643 0.284008 0.284008 0.284008 0.293139 0.293139 0.293139 0.302047 0.302047 0.302047 0.310743 0.310743 0.310743 0.319241 0.319241 0.319241 0.327556 0.327556 0.327556 0.335706 0.335706 0.335706 0.343713 0.343713 0.343713 0.351599 0.351599 0.351599 0.359392 0.359392 0.359392 0.367126 0.367126 0.367126 0.374835 0.374835 0.374835 0.382562 0.382562 0.382562 0.390352 0.390352 0.390352 0.398256 0.398256 0.398256 0.406325 0.406325 0.406325 0.41461 0.41461 0.41461 0.423156 0.423156 0.423156 0.431994 0.431994 0.431994 0.441132 0.441132 0.441132 0.450548 0.450548 0.450548 0.460189 0.460189 0.460189 0.467051 0.467051 0.467051 0.5 0.5 0.5 0.532949 0.532949 0.532949 0.539811 0.539811 0.539811 0.549452 0.549452 0.549452 0.558868 0.558868 0.558868 0.568006 0.568006 0.568006 0.576844 0.576844 0.576844 0.58539 0.58539 0.58539 0.593675 0.593675 0.593675 0.601744 0.601744 0.601744 0.609648 0.609648 0.609648 0.617438 0.617438 0.617438 0.625165 0.625165 0.625165 0.632874 0.632874 0.632874 0.640608 0.640608 0.640608 0.648401 0.648401 0.648401 0.656287 0.656287 0.656287 0.664294 0.664294 0.664294 0.672444 0.672444 0.672444 0.680759 0.680759 0.680759 0.689257 0.689257 0.689257 0.697953 0.697953 0.697953 0.706861 0.706861 0.706861 0.715992 0.715992 0.715992 0.725357 0.725357 0.725357 0.734965 0.734965 0.734965 0.744824 0.744824 0.744824 0.75494 0.75494 0.75494 0.765319 0.765319 0.765319 0.777716 0.777716 0.777716 0.794089 0.794089 0.794089 0.802889 0.802889 0.802889 0.812862 0.812862 0.812862 0.824009 0.824009 0.824009 0.836328 0.836328 0.836328 0.849822 0.849822 0.849822 0.864488 0.864488 0.864488 0.880328 0.880328 0.880328 0.897341 0.897341 0.897341 0.915527 0.915527 0.915527 0.934887 0.934887 0.934887 1 1 1 1
  arc A272 (-45.5054, 85.4178) -> (-46.5003, 85.3932) centre (-45.7832, 76.5321) ccw
  spline S71 degree 3 poles (-49.9854, 84.3663) (-49.8491, 84.2941) (-49.716, 84.2157) (-49.5876, 84.1302) (-49.5494, 84.1048) (-49.5117, 84.0787) (-49.4744, 84.052) (-49.4393, 84.027) (-49.4047, 84.0013) (-49.3705, 83.9751) (-49.3385, 83.9506) (-49.3069, 83.9255) (-49.2758, 83.8999) (-49.2468, 83.8761) (-49.2182, 83.8518) (-49.1901, 83.827) (-49.164, 83.804) (-49.1383, 83.7806) (-49.113, 83.7568) (-49.0897, 83.7349) (-49.0668, 83.7126) (-49.0443, 83.6899) (-49.0237, 83.6692) (-49.0035, 83.6482) (-48.9836, 83.6268) (-48.9657, 83.6074) (-48.9481, 83.5877) (-48.9307, 83.5678) (-48.9151, 83.55) (-48.8998, 83.532) (-48.8851, 83.5135) (-48.8722, 83.4972) (-48.8599, 83.4806) (-48.8466, 83.4643) (-48.8218, 83.4339) (-48.7933, 83.4044) (-48.7801, 83.3688) (-48.7701, 83.3418) (-48.7687, 83.3114) (-48.7642, 83.2821) (-48.7604, 83.2576) (-48.7544, 83.2339) (-48.7485, 83.2101) (-48.7428, 83.1868) (-48.7372, 83.1635) (-48.7311, 83.1403) (-48.7252, 83.1177) (-48.7188, 83.0952) (-48.7121, 83.0729) (-48.7056, 83.0511) (-48.6987, 83.0293) (-48.6915, 83.0078) (-48.6845, 82.9867) (-48.6771, 82.9658) (-48.6694, 82.945) (-48.6618, 82.9247) (-48.654, 82.9046) (-48.6457, 82.8846) (-48.6377, 82.8651) (-48.6293, 82.8457) (-48.6206, 82.8265) (-48.612, 82.8077) (-48.6032, 82.7891) (-48.5939, 82.7707) (-48.5849, 82.7527) (-48.5755, 82.7349) (-48.5658, 82.7173) (-48.5563, 82.7) (-48.5464, 82.6829) (-48.5362, 82.6661) (-48.5262, 82.6496) (-48.5158, 82.6333) (-48.5051, 82.6173) (-48.4945, 82.6015) (-48.4836, 82.586) (-48.4724, 82.5707) (-48.4613, 82.5557) (-48.4498, 82.5409) (-48.438, 82.5264) (-48.4263, 82.5121) (-48.4143, 82.4981) (-48.4019, 82.4845) (-48.3895, 82.4709) (-48.3768, 82.4577) (-48.3638, 82.4448) (-48.3507, 82.432) (-48.3373, 82.4196) (-48.3236, 82.4076) (-48.3098, 82.3956) (-48.2956, 82.384) (-48.281, 82.3729) (-48.2663, 82.3617) (-48.2512, 82.3511) (-48.2358, 82.341) (-48.2201, 82.3307) (-48.2041, 82.321) (-48.1877, 82.312) (-48.1709, 82.3028) (-48.1538, 82.2942) (-48.1363, 82.2864) (-48.1184, 82.2784) (-48.1001, 82.2712) (-48.0815, 82.2649) (-48.0624, 82.2583) (-48.0429, 82.2527) (-48.0232, 82.2481) (-48.0028, 82.2433) (-47.9821, 82.2396) (-47.9614, 82.237) (-47.9399, 82.2343) (-47.9182, 82.2328) (-47.8966, 82.2326) (-47.8742, 82.2324) (-47.8519, 82.2335) (-47.8297, 82.236) (-47.807, 82.2385) (-47.7845, 82.2425) (-47.7622, 82.2477) (-47.7464, 82.2515) (-47.7307, 82.2558) (-47.7151, 82.2603) (-47.6402, 82.2822) (-47.5667, 82.3088) (-47.4918, 82.3309) (-47.417, 82.3529) (-47.3408, 82.3704) (-47.266, 82.3927) (-47.2504, 82.3973) (-47.2349, 82.4022) (-47.2196, 82.4076) (-47.198, 82.4153) (-47.1769, 82.4242) (-47.1564, 82.4343) (-47.1365, 82.4443) (-47.1171, 82.4555) (-47.0985, 82.4678) (-47.0804, 82.4797) (-47.063, 82.4927) (-47.0464, 82.5066) (-47.0303, 82.52) (-47.015, 82.5343) (-47.0005, 82.5494) (-46.9864, 82.564) (-46.9731, 82.5793) (-46.9605, 82.5952) (-46.9484, 82.6106) (-46.9369, 82.6266) (-46.9262, 82.643) (-46.9157, 82.659) (-46.906, 82.6755) (-46.8969, 82.6923) (-46.888, 82.7088) (-46.8798, 82.7256) (-46.8722, 82.7427) (-46.8647, 82.7596) (-46.8578, 82.7768) (-46.8515, 82.7941) (-46.8453, 82.8113) (-46.8397, 82.8288) (-46.8346, 82.8464) (-46.8295, 82.8639) (-46.825, 82.8816) (-46.821, 82.8994) (-46.817, 82.9173) (-46.8135, 82.9353) (-46.8105, 82.9534) (-46.8074, 82.9716) (-46.8049, 82.9899) (-46.8029, 83.0082) (-46.8008, 83.0268) (-46.7991, 83.0454) (-46.798, 83.0641) (-46.7968, 83.083) (-46.796, 83.102) (-46.7957, 83.1209) (-46.7954, 83.1402) (-46.7955, 83.1595) (-46.7961, 83.1788) (-46.7966, 83.1985) (-46.7976, 83.2182) (-46.7989, 83.2379) (-46.8003, 83.258) (-46.8021, 83.278) (-46.8043, 83.298) (-46.8065, 83.3185) (-46.8092, 83.3389) (-46.8122, 83.3593) (-46.8152, 83.3802) (-46.8187, 83.401) (-46.8225, 83.4218) (-46.8264, 83.443) (-46.8307, 83.4643) (-46.8354, 83.4854) (-46.8402, 83.507) (-46.8453, 83.5286) (-46.8508, 83.5501) (-46.8565, 83.5722) (-46.8625, 83.5941) (-46.8688, 83.616) (-46.8753, 83.6384) (-46.8821, 83.6608) (-46.8894, 83.683) (-46.8969, 83.7057) (-46.9048, 83.7284) (-46.9126, 83.751) (-46.9206, 83.7742) (-46.9284, 83.7974) (-46.9385, 83.8201) (-46.9506, 83.8471) (-46.966, 83.8734) (-46.9722, 83.9015) (-46.9803, 83.9386) (-46.9725, 83.9788) (-46.9681, 84.0178) (-46.9657, 84.0388) (-46.9644, 84.0594) (-46.9624, 84.0801) (-46.9601, 84.1035) (-46.9569, 84.127) (-46.9535, 84.1504) (-46.9497, 84.1766) (-46.9456, 84.2026) (-46.941, 84.2286) (-46.936, 84.2574) (-46.9304, 84.286) (-46.9243, 84.3146) (-46.9177, 84.3458) (-46.9105, 84.377) (-46.9029, 84.408) (-46.8945, 84.4418) (-46.8856, 84.4753) (-46.8761, 84.5088) (-46.8659, 84.5449) (-46.8551, 84.5808) (-46.8436, 84.6166) (-46.8314, 84.6549) (-46.8184, 84.6931) (-46.8049, 84.7311) (-46.7904, 84.7716) (-46.7752, 84.812) (-46.7593, 84.852) (-46.7424, 84.8947) (-46.7248, 84.937) (-46.7065, 84.9791) (-46.645, 85.1205) (-46.5757, 85.2586) (-46.5003, 85.3932) knots 0 0 0 0 0.065113 0.065113 0.065113 0.084473 0.084473 0.084473 0.102659 0.102659 0.102659 0.119672 0.119672 0.119672 0.135512 0.135512 0.135512 0.150178 0.150178 0.150178 0.163672 0.163672 0.163672 0.175991 0.175991 0.175991 0.187138 0.187138 0.187138 0.197111 0.197111 0.197111 0.205911 0.205911 0.205911 0.222284 0.222284 0.222284 0.234681 0.234681 0.234681 0.24506 0.24506 0.24506 0.255176 0.255176 0.255176 0.265035 0.265035 0.265035 0.274643 0.274643 0.274643 0.284008 0.284008 0.284008 0.293139 0.293139 0.293139 0.302047 0.302047 0.302047 0.310743 0.310743 0.310743 0.319241 0.319241 0.319241 0.327556 0.327556 0.327556 0.335706 0.335706 0.335706 0.343713 0.343713 0.343713 0.351599 0.351599 0.351599 0.359392 0.359392 0.359392 0.367126 0.367126 0.367126 0.374835 0.374835 0.374835 0.382562 0.382562 0.382562 0.390352 0.390352 0.390352 0.398256 0.398256 0.398256 0.406325 0.406325 0.406325 0.41461 0.41461 0.41461 0.423156 0.423156 0.423156 0.431994 0.431994 0.431994 0.441132 0.441132 0.441132 0.450548 0.450548 0.450548 0.460189 0.460189 0.460189 0.467051 0.467051 0.467051 0.5 0.5 0.5 0.532949 0.532949 0.532949 0.539811 0.539811 0.539811 0.549452 0.549452 0.549452 0.558868 0.558868 0.558868 0.568006 0.568006 0.568006 0.576844 0.576844 0.576844 0.58539 0.58539 0.58539 0.593675 0.593675 0.593675 0.601744 0.601744 0.601744 0.609648 0.609648 0.609648 0.617438 0.617438 0.617438 0.625165 0.625165 0.625165 0.632874 0.632874 0.632874 0.640608 0.640608 0.640608 0.648401 0.648401 0.648401 0.656287 0.656287 0.656287 0.664294 0.664294 0.664294 0.672444 0.672444 0.672444 0.680759 0.680759 0.680759 0.689257 0.689257 0.689257 0.697953 0.697953 0.697953 0.706861 0.706861 0.706861 0.715992 0.715992 0.715992 0.725357 0.725357 0.725357 0.734965 0.734965 0.734965 0.744824 0.744824 0.744824 0.75494 0.75494 0.75494 0.765319 0.765319 0.765319 0.777716 0.777716 0.777716 0.794089 0.794089 0.794089 0.802889 0.802889 0.802889 0.812862 0.812862 0.812862 0.824009 0.824009 0.824009 0.836328 0.836328 0.836328 0.849822 0.849822 0.849822 0.864488 0.864488 0.864488 0.880328 0.880328 0.880328 0.897341 0.897341 0.897341 0.915527 0.915527 0.915527 0.934887 0.934887 0.934887 1 1 1 1
  arc A273 (-49.9854, 84.3663) -> (-50.8347, 83.8475) centre (-45.7832, 76.5321) ccw
  line L62 (-44.9072, 81.5554) -> (-44.8793, 80.4287)
  arc A274 (-46.8787, 80.3792) -> (-44.8793, 80.4287) centre (-45.7832, 76.5321) ccw
  line L63 (-46.9066, 81.5059) -> (-46.8787, 80.3792)
  line L64 (-44.9072, 81.5554) -> (-46.9066, 81.5059)